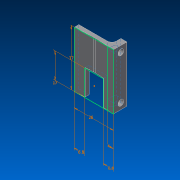
# Autodesk Inventor part: psu rear brace
Saved by Autodesk Inventor 2015 (Build 190159000, 159)
## iProperties
Created: 2017-03-20
Part Number: psu rear brace
Material: Generic
Document SubType Name: Modeling
Designer: ZigZagJoe
Density: 1 g/cm^3
Appearance: Default
Author: ZigZagJoe
Autodesk Inventor part; units mm, degrees
ref_plane "YZ Plane" through (0, 0, 0) normal (1, 0, 0) x (0, 1, 0)
ref_plane "XZ Plane" through (0, 0, 0) normal (0, 1, 0) x (-1, 0, 0)
ref_plane "XY Plane" through (0, 0, 0) normal (0, 0, 1) x (1, 0, 0)
sketch "Sketch1" plane through (0, 0, 0) normal (0, 1, 0) x (-1, 0, 0)
  line L0 (13.3302, 27.1778) -> (-12.6698, 27.1778)
  line L1 (-12.6698, 27.1778) -> (-12.6698, -9.8222)
  line L2 (-12.6698, -9.8222) -> (13.3302, -9.8222)
  line L3 (13.3302, -9.8222) -> (13.3302, 27.1778)
  line L4 (6.5302, 7.1778) -> (-5.8698, 7.1778)
  line L5 (-5.8698, 7.1778) -> (-5.8698, -9.8222)
  line L6 (-5.8698, -9.8222) -> (6.5302, -9.8222)
  line L7 (6.5302, -9.8222) -> (6.5302, 7.1778)
  line L8 (-12.6698, 27.1778) -> (-8.6698, 27.1778)
  line L9 (-8.6698, 27.1778) -> (-8.6698, -9.8222)
  line L10 (-8.6698, -9.8222) -> (-12.6698, -9.8222)
  line L11 (-12.6698, -9.8222) -> (-12.6698, 27.1778)
  point P0 (0, 0)
  dimension "d0" = 26
  dimension "d1" = 37
  dimension "d2" = 6.8
  dimension "d3" = 6.8
  dimension "d4" = 17
  dimension "d5" = 4
  constraints: 24 end point, 6 parallel, 3 horizontal, 3 perpendicular, 2 point on line
  measures "d0" distance of L1.end L2.end
  measures "d1" distance of L2.end L0.start
  measures "d2" distance between parallel lines of L3 L7
  measures "d3" distance between parallel lines of L1 L5
  measures "d4" distance of L6.end L4.start
  measures "d5" distance between parallel lines of L1 L9
extrude "Extrusion1" add sketch "Sketch1" along normal blind 3 contours L3 L2 L7 L4 L5 L9 L0 | L9 L2 L1 L0
extrude "Extrusion2" add sketch "Sketch1" along normal blind 9 contours L9 L2 L1 L0
sketch "Sketch2" plane through (12.6698, 0, 27.1778) normal (1, 0, 0) x (0, 0, -1)
  circle A0 centre (4, 5) radius 1.9
  circle A1 centre (33, 5) radius 1.9
  line L0 (0, 0) -> (0, 9) projected
  line L1 (37, 0) -> (37, 9) projected
  line L2 (0, 0) -> (37, 0) projected
  point P0 (27.1778, 0)
  dimension "d10" = 3.8
  dimension "d11" = 3.8
  dimension "d12" = 4
  dimension "d13" = 4
  dimension "d14" = 4
  dimension "d15" = 4
  dimension "d27" = 5
  dimension "d28" = 29
  constraints: 2 centre point
  measures "d10" diameter of A0
  measures "d11" diameter of A1
  measures "d12" distance from line of L0 A0.centre
  measures "d13" distance from line of L1 A1.centre
  measures "d14" horizontal distance of L0.end A0.centre
  measures "d15" horizontal distance of A1.centre L1.end
  measures "d27" distance from line of L2 A0.centre
  measures "d28" distance of A1.centre A0.centre
extrude "Extrusion3" cut sketch "Sketch2" against normal blind 8
fillet "Fillet1" radius 3 1 edges at (8.6698, 3, 8.6778)
sketch "Sketch3" plane through (-13.3302, 0, 27.1778) normal (0, 0, 1) x (1, 0, 0)
  line L0 (26, 0) -> (13.75, 0.65)
  line L1 (12.25, 0.65) -> (0, 0)
  line L2 (0, 0) -> (26, 0)
  line L3 (0, 0) -> (26, 0) projected
  line L4 (0, 0) -> (0, 3) projected
  line L5 (26, 0) -> (26, 9) projected
  line L6 (13.75, 0.65) -> (12.25, 0.65)
  point P0 (13.3302, 0)
  dimension "d21" = 26
  dimension "d24" = 0.65
  dimension "d25" = 1.5
  dimension "d26" = 12.25
  constraints: 8 end point, 1 collinear, 1 horizontal, 1 parallel
  measures "d21" distance between parallel lines of L5 L4
  measures "d24" distance between parallel lines of L2 L6
  measures "d25" distance of L1.start L0.end
  measures "d26" distance from line of L5 L0.end
extrude "Extrusion4" cut sketch "Sketch3" against normal blind 40
equation "\"d26\" = 0.5 * d21 - 0.5 * d25"
body "Solid1"
